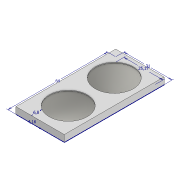
# Autodesk Inventor part: ShelfLabel
Saved by Autodesk Inventor 2020.3 (Build 243373000, 373)
## iProperties
Created: 2021-08-20
Part Number: ShelfLabel
Material: Generic
Document SubType Name: Modeling
Designer: Yusuf
Mass: 5.85188 g
Surface Area: 51.255 cm^2
Volume: 5.85188 cm^3
Density: 1 g/cm^3
Appearance: Default
Author: Yusuf
Autodesk Inventor part; units mm, degrees
ref_plane "YZ Plane" through (0, 0, 0) normal (1, 0, 0) x (0, 1, 0)
ref_plane "XZ Plane" through (0, 0, 0) normal (0, 1, 0) x (-1, 0, 0)
ref_plane "XY Plane" through (0, 0, 0) normal (0, 0, 1) x (1, 0, 0)
sketch "Sketch1" plane through (0, 0, 0) normal (0, 1, 0) x (-1, 0, 0)
  line L0 (0, 0) -> (31, 0)
  line L1 (31, 0) -> (31, -64)
  line L2 (31, -64) -> (0, -64)
  line L3 (0, -64) -> (0, 0)
  line L4 (28.085, -10.96) -> (2.915, -10.96)
  line L5 (2.915, -10.96) -> (2.915, -61.085)
  line L6 (2.915, -61.085) -> (28.085, -61.085)
  line L7 (28.085, -61.085) -> (28.085, -10.96)
  line L8 (31, -43.4956) -> (28.085, -43.4956) construction
  line L9 (15.5, -61.085) -> (15.5, -64) construction
  line L10 (31, -4.16) -> (0, -4.16)
  line L11 (31, -10.96) -> (0, -10.96)
  point P0 (15.5, -10.96)
  point P1 (15.5, 0)
  dimension "d0" = 31
  dimension "d1" = 64
  dimension "d2" = 25.17
  dimension "d4" = 4.16
  dimension "d5" = 6.8
  constraints: 24 end point, 6 perpendicular, 6 point on line, 5 midpoint, 4 parallel, 2 horizontal, 1 vertical alignment
  measures "d0" distance of L1.end L2.end
  measures "d1" distance of L0.end L1.end
  measures "d2" distance of L6.end L5.end
  measures "d4" distance between parallel lines of L0 L10
  measures "d5" distance between parallel lines of L11 L10
extrude "Extrusion1" add sketch "Sketch1" along normal blind 4.3
extrude "Extrusion2" cut sketch "Sketch1" along normal blind 1.75 contours L4 L7 L6 L5
sketch "Sketch2" plane through (0, 4.3, 0) normal (0, 1, 0) x (1, 0, 0)
  circle A0 centre (-15.5, 47.57) radius 12.25
  line L0 (0, 64) -> (-31, 64) projected
  circle A1 centre (-14.7283, 17.25) radius 12.25
  line L1 (-31, 0) -> (0, 0) projected
  point P0 (-15.5, 64)
  dimension "d10" = 24.5
  dimension "d11" = 4.18
  dimension "d13" = 29.5
  constraints: 2 centre point, 1 equal radius, 1 midpoint, 1 vertical alignment
  measures "d10" diameter of A0
  measures "d11" distance edge to line of A0 L0
extrude "Extrusion3" cut sketch "Sketch2" against normal blind 0.5
body "Solid1"
